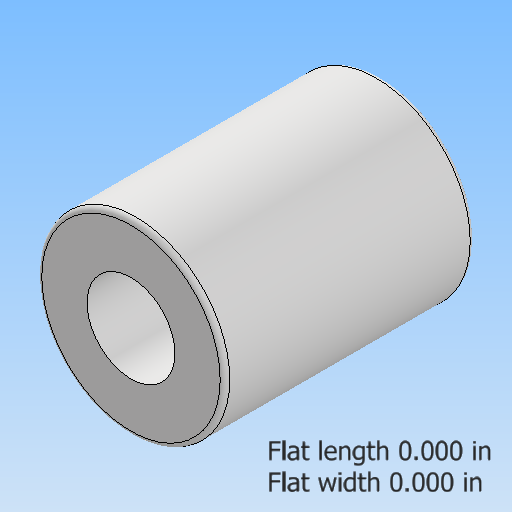
# Autodesk Inventor part: Shaft Coupler
Saved by Autodesk Inventor 2025.4 (Build 294407000, 407)
## iProperties
RuleStatus: InUse
Created: 2025-09-16
Part Number: Shaft Coupler
Material: Steel, Mild
Document SubType Name: Modeling
Designer: josh
Mass: 790.626 g
Surface Area: 2648.86 cm^2
Volume: 295.01 cm^3
Density: 7.85 g/cm^3
Sheet Metal Rule: Mild Steel .188
Sheet Metal Width: 0.000 in
Sheet Metal Length: 0.000 in
Sheet Metal Area: 0.000 in^2
Appearance: Default
Description: Brush Roller to Drive Connector Bushing
AfterDocOpen0: PartNumber
Flat pattern length: =<Sheet Metal Length>
Flat pattern width: =<Sheet Metal Width>
Thickness: 0.188 in
Qty: 1
Flat Length: 0.0
Flat Width: 0.0
Part Area: 0.0
Author: josh
Autodesk Inventor part; units mm, degrees
ref_plane "YZ Plane" through (0, 0, 0) normal (1, 0, 0) x (0, 1, 0)
ref_plane "XZ Plane" through (0, 0, 0) normal (0, 1, 0) x (-1, 0, 0)
ref_plane "XY Plane" through (0, 0, 0) normal (0, 0, 1) x (1, 0, 0)
sketch "Sketch12" plane through (0, 0, 0) normal (0, 0, 1) x (1, 0, 0)
  circle A0 centre (0, 0) radius 14.986
  circle A1 centre (0, 0) radius 5
  dimension "d107" = 29.972
  dimension "d108" = 10
  constraints: 2 centre point, 2 coincident
  measures "d107" diameter of A0
  measures "d108" diameter of A1
extrude "Extrusion1" add sketch "Sketch12" along normal mid plane 39.878
sketch "Sketch13" plane through (0, 0, 19.939) normal (0, 0, 1) x (1, 0, 0)
  circle A0 centre (0, 0) radius 5 construction
  circle A1 centre (0, 0) radius 7.0104
  dimension "d111" = 14.0208
  constraints: 1 centre point, 1 coincident
  measures "d111" diameter of A1
extrude "Extrusion2" cut sketch "Sketch13" against normal blind 19.939
fillet "Fillet1" radius 0.762 2 edges at (-14.986, 0, -19.939) (-14.986, 0, 19.939)
equation "\"BendRadius\" = Thickness"
equation "\"BendReliefWidth\" = Thickness"
equation "\"BendReliefDepth\" = 0.5 * Thickness"
equation "\"CornerReliefSize\" = 4 * Thickness"
equation "\"MinimumRemnant\" = 2 * Thickness"
equation "\"TransitionRadius\" = BendRadius"
equation "\"JacobiRadiusSize\" = BendRadius"
equation "\"GapSize\" = Thickness"
equation "\"Thickness\" = 4.7625"
body "Solid3"
